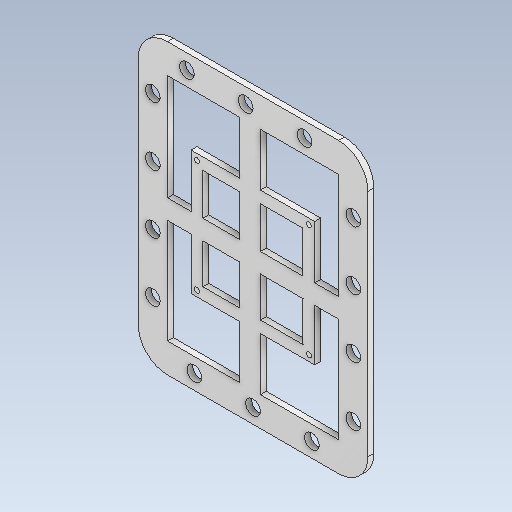
# Autodesk Inventor part: top
Saved by Autodesk Inventor 2020 (Build 240168000, 168)
## iProperties
Created: 2019-06-14
Part Number: top
Material: ABS Plastic
Document SubType Name: Modeling
Designer: amirt
Density: 1.06 g/cm^3
Appearance: Smooth - White
Author: amirt
Autodesk Inventor part; units mm, degrees
ref_plane "YZ Plane" through (0, 0, 0) normal (1, 0, 0) x (0, 1, 0)
ref_plane "XZ Plane" through (0, 0, 0) normal (0, 1, 0) x (-1, 0, 0)
ref_plane "XY Plane" through (0, 0, 0) normal (0, 0, 1) x (1, 0, 0)
sketch "Sketch1" plane through (0, 0, 0) normal (0, 0, 1) x (1, 0, 0)
  line L0 (-25.4, 0) -> (-25.4, 25.4)
  line L1 (-25.4, 25.4) -> (0, 25.4)
  circle A0 centre (48.4909, -48.4909) radius 1.1 projected
  line L2 (73.8909, -48.4909) -> (73.8909, -73.8909)
  line L3 (73.8909, -73.8909) -> (48.4909, -73.8909)
  line L4 (73.8909, -73.8909) -> (-25.4, -73.8909)
  line L5 (-25.4, -73.8909) -> (-25.4, 25.4)
  line L6 (-25.4, 25.4) -> (73.8909, 25.4)
  line L7 (73.8909, 25.4) -> (73.8909, -73.8909)
  line L8 (73.8909, -73.8909) -> (-25.4, -73.8909)
  line L9 (-25.4, -73.8909) -> (-25.4, -61.1909)
  line L10 (73.8909, -61.1909) -> (73.8909, -73.8909)
  line L11 (73.8909, 25.4) -> (-25.4, 25.4)
  line L12 (-25.4, 25.4) -> (-25.4, 12.7)
  line L13 (73.8909, 12.7) -> (73.8909, 25.4)
  line L14 (-25.4, -73.8909) -> (-12.7, -73.8909)
  line L15 (-12.7, 25.4) -> (-25.4, 25.4)
  line L16 (-25.4, 25.4) -> (-25.4, -73.8909)
  line L17 (73.8909, -73.8909) -> (61.1909, -73.8909)
  line L18 (61.1909, 25.4) -> (73.8909, 25.4)
  line L19 (73.8909, 25.4) -> (73.8909, -73.8909)
  line L20 (-12.7, -73.8909) -> (61.1909, -73.8909)
  line L21 (61.1909, -73.8909) -> (61.1909, -86.5909)
  line L22 (61.1909, -86.5909) -> (-12.7, -86.5909)
  line L23 (-12.7, -86.5909) -> (-12.7, -73.8909)
  line L24 (61.1909, 25.4) -> (-12.7, 25.4)
  line L25 (-12.7, 25.4) -> (-12.7, 38.1)
  line L26 (-12.7, 38.1) -> (61.1909, 38.1)
  line L27 (61.1909, 38.1) -> (61.1909, 25.4)
  line L28 (61.1909, -73.8909) -> (61.1909, 25.4)
  line L29 (-12.7, 25.4) -> (-12.7, -73.8909)
  circle A1 centre (-1.1557, -80.2409) radius 3.175
  circle A2 centre (24.2443, -80.2409) radius 3.175
  circle A3 centre (49.6443, -80.2409) radius 3.175
  circle A4 centre (-4.3307, 31.6283) radius 3.175
  circle A5 centre (21.0693, 31.6283) radius 3.175
  circle A6 centre (46.4693, 31.6283) radius 3.175
  circle A7 centre (-19.05, 15.5507) radius 3.175
  circle A8 centre (-19.05, -9.8493) radius 3.175
  circle A9 centre (-19.05, -35.2493) radius 3.175
  circle A10 centre (-19.05, -60.6493) radius 3.175
  circle A11 centre (67.5409, 12.3757) radius 3.175
  circle A12 centre (67.5409, -13.0243) radius 3.175
  circle A13 centre (67.5409, -38.4243) radius 3.175
  circle A14 centre (67.5409, -63.8243) radius 3.175
  line L30 (27.4193, -73.8909) -> (18.4699, -73.8909)
  line L31 (18.4699, -73.8909) -> (18.4699, 25.4)
  line L32 (18.4699, 25.4) -> (27.4193, 25.4)
  line L33 (27.4193, 25.4) -> (27.4193, -73.8909)
  line L34 (-12.7, -28.772) -> (61.1909, -28.772)
  line L35 (61.1909, -28.772) -> (61.1909, -20.3296)
  line L36 (61.1909, -20.3296) -> (-12.7, -20.3296)
  line L37 (-12.7, -20.3296) -> (-12.7, -28.772)
  arc A15 (-25.4, -73.8909) -> (-12.7, -86.5909) centre (-12.7, -73.8909) ccw
  arc A16 (61.1909, -86.5909) -> (73.8909, -73.8909) centre (61.1909, -73.8909) ccw
  arc A17 (-12.7, 38.1) -> (-25.4, 25.4) centre (-12.7, 25.4) ccw
  arc A18 (73.8909, 25.4) -> (61.1909, 38.1) centre (61.1909, 25.4) ccw
  circle A19 centre (0, -48.4909) radius 1.1 projected
  circle A20 centre (0, 0) radius 1.1 projected
  circle A21 centre (48.3594, 0.0969) radius 1.1 projected
  circle A22 centre (48.4909, -48.4909) radius 1.1 projected
  line L38 (-2.54, -51.0309) -> (50.8994, -51.0309)
  line L39 (50.8994, -51.0309) -> (50.8994, 2.6369)
  line L40 (50.8994, 2.6369) -> (-2.54, 2.6369)
  line L41 (-2.54, 2.6369) -> (-2.54, -51.0309)
  line L42 (2.54, -45.9509) -> (45.8194, -45.9509)
  line L43 (45.8194, -45.9509) -> (45.8194, -2.4431)
  line L44 (45.8194, -2.4431) -> (2.54, -2.4431)
  line L45 (2.54, -2.4431) -> (2.54, -45.9509)
  point P0 (0, 0)
  point P1 (24.2455, -24.2455)
  point P2 (27.4193, -20.3296)
  point P3 (18.4699, -20.3296)
  point P4 (-12.7, -20.3296)
  point P5 (18.4699, -28.772)
  point P6 (27.4193, -28.772)
  point P7 (45.8194, -28.772)
  point P8 (27.4193, -45.9509)
  point P9 (27.4193, -51.0309)
  point P10 (50.8994, -28.772)
  point P11 (27.4193, -2.4431)
  point P12 (45.8194, -20.3296)
  point P13 (50.8994, -20.3296)
  point P14 (27.4193, 2.6369)
  point P15 (2.54, -20.3296)
  point P16 (18.4699, -2.4431)
  point P17 (18.4699, 2.6369)
  point P18 (-2.54, -20.3296)
  point P19 (2.54, -28.772)
  point P20 (-2.54, -28.772)
  point P21 (18.4699, -51.0309)
  point P22 (18.4699, -45.9509)
  dimension "d0" = 25.4
  dimension "d1" = 25.4
  dimension "d2" = 25.4
  dimension "d3" = 25.4
  dimension "d4" = 12.7
  dimension "d5" = 12.7
  dimension "d6" = 12.7
  dimension "d7" = 12.7
  dimension "d8" = 12.7
  dimension "d9" = 12.7
  dimension "d10" = 6.35
  dimension "d11" = 11.5443
  dimension "d14" = 25.4
  dimension "d21" = 6.35
  dimension "d24" = 25.4
  dimension "d29" = 6.35
  dimension "d32" = 25.4
  dimension "d37" = 6.35
  dimension "d40" = 25.4
  constraints: 92 end point, 19 parallel, 18 centre point, 11 horizontal, 10 perpendicular, 9 point on line, 8 point on circle, 8 tangent, 2 vertical, 20 other
  measures "d0" distance of L0.end L1.end
  measures "d1" distance of L0.start L0.end
  measures "d2" distance of L2.end L3.end
  measures "d3" distance of L2.start L2.end
  measures "d4" distance of L8.end L9.end
  measures "d5" distance of L12.end L11.end
  measures "d6" distance of L15.end L15.start
  measures "d7" distance of L18.start L18.end
  measures "d8" distance of L20.end L21.end
  measures "d9" distance of L24.end L25.end
  measures "d10" diameter of A1
  measures "d11" distance from line of L23 A1.centre
  measures "d14" distance of A1.centre A2.centre
  measures "d21" diameter of A4
  measures "d24" distance of A4.centre A5.centre
  measures "d29" diameter of A7
  measures "d32" distance of A7.centre A8.centre
  measures "d37" diameter of A11
  measures "d40" distance of A11.centre A12.centre
extrude "Extrusion1" add sketch "Sketch1" along normal blind 2.54 contours L0 L1 L29 L4 L5 | A17 L25 L1 | L4 L23 A15 | L25 L26 L27 L6 L1 | L4 L3 L21 L22 L23 | L36 L41 L34 L29 | A18 L6 L27 | L31 L38 L33 L4 | L21 L3 A16 | L6 L33 L40 L31 | L41 L40 L31 L44 L45 L36 | L36 L45 L34 L41 | L6 L7 L2 L3 L28 | L38 L41 L34 L45 L42 L31 | L31 L42 L33 L38 | L40 L33 L44 L31 | L36 L31 L34 L45 | L28 L34 L39 L36 | L33 L42 L43 L34 L39 L38 | L31 L34 L33 L42 | L40 L39 L36 L43 L44 L33 | L44 L33 L36 L31 | L36 L33 L34 L31 | L39 L34 L43 L36 | L36 L43 L34 L33
body "Solid1"
